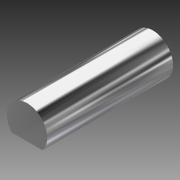
# Autodesk Inventor part: Motor Shaft
Saved by Autodesk Inventor 2014 (Build 180170000, 170)
## iProperties
Created: 2014-02-03
Part Number: Motor Shaft
Material: Generic
Document SubType Name: Modeling
Designer: Spooner
Density: 1 g/cm^3
Appearance: Chrome - Polished
Author: Spooner
Autodesk Inventor part; units mm, degrees
ref_plane "YZ Plane" through (0, 0, 0) normal (1, 0, 0) x (0, 1, 0)
ref_plane "XZ Plane" through (0, 0, 0) normal (0, 1, 0) x (-1, 0, 0)
ref_plane "XY Plane" through (0, 0, 0) normal (0, 0, 1) x (1, 0, 0)
sketch "Sketch1" plane through (0, 0, 0) normal (0, 0, 1) x (1, 0, 0)
  circle A0 centre (0, 0) radius 1.9304
  dimension "d0" = 3.8608
  constraints: 1 centre point, 1 coincident
  measures "d0" diameter of A0
extrude "Extrusion1" add sketch "Sketch1" along normal blind 12.065
sketch "Sketch2" plane through (0, 0, 12.065) normal (0, 0, 1) x (1, 0, 0)
  circle A0 centre (0, 0) radius 1.9304 projected
  line L0 (-1.4756, -1.2446) -> (1.4756, -1.2446)
  dimension "d3" = 3.175
  constraints: 2 end point, 2 point on circle, 1 horizontal
extrude "Extrusion2" cut sketch "Sketch2" against normal blind 6.604 contours L0 A0 picked at (-0.3747, -1.3529)
body "Solid1"
